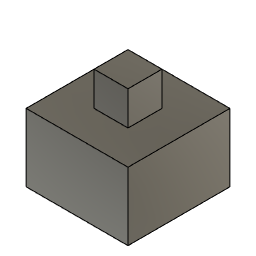
1x1Block (Autodesk Fusion 360 design; units mm, degrees)
Autodesk Fusion 360 part; units mm, degrees
sketch "Sketch2" plane through (0, 0, 0) normal (0, 0, 1) x (1, 0, 0)
  line L0 (0, 0) -> (15, 0)
  line L1 (15, 0) -> (15, 15)
  line L2 (15, 15) -> (0, 15)
  line L3 (0, 15) -> (0, 0)
  line L4 (5, 10) -> (10, 10)
  line L5 (10, 10) -> (10, 5)
  line L6 (10, 5) -> (5, 5)
  line L7 (5, 5) -> (5, 10)
  line L8 (4.825, 10.175) -> (10.175, 10.175)
  line L9 (10.175, 10.175) -> (10.175, 4.825)
  line L10 (10.175, 4.825) -> (4.825, 4.825)
  line L11 (4.825, 4.825) -> (4.825, 10.175)
  dimension "d5" = -0.175
  constraint horizontal L0
  constraint vertical L1
  constraint horizontal L2
  constraint vertical L3
  constraint coincident L0.start L3.end
  constraint horizontal L4
  constraint vertical L5
  constraint horizontal L6
  constraint vertical L7
extrude "Extrude1" add sketch "Sketch2" along normal blind 10 contours L0 L1 L2 L3 | L8 L9 L10 L11
extrude "Extrude2" add sketch "Sketch2" along normal blind 15 contours L4 L5 L6 L7
extrude "Extrude3" cut sketch "Sketch2" along normal blind 6.175 contours L4 L5 L6 L7 | L8 L9 L10 L11
extrude "Extrude4" add 1 faces at (8.3917, 8.3917, 6.175) along direction (0, 0, -1) blind 1
